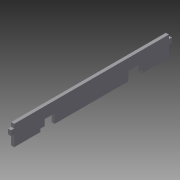
# Autodesk Inventor part: MainPanelWall3
Saved by Autodesk Inventor 2015 (Build 190159000, 159)
## iProperties
Created: 2014-08-06
Part Number: MainPanelWall3
Material: Generic
Document SubType Name: Modeling
Designer: STACKPOLE
Density: 1 g/cm^3
Appearance: Default
Author: STACKPOLE
Autodesk Inventor part; units mm, degrees
ref_plane "YZ Plane" through (0, 0, 0) normal (1, 0, 0) x (0, 1, 0)
ref_plane "XZ Plane" through (0, 0, 0) normal (0, 1, 0) x (-1, 0, 0)
ref_plane "XY Plane" through (0, 0, 0) normal (0, 0, 1) x (1, 0, 0)
sketch "Sketch1" plane through (0, 0, 0) normal (1, 0, 0) x (0, 1, 0)
  line L0 (0, 11) -> (-3, 11)
  line L1 (-3, 11) -> (-3, 16)
  line L2 (-3, 16) -> (0, 16)
  line L3 (0, 20) -> (0, 16)
  line L4 (0, 11) -> (0, 0)
  line L5 (153, 16) -> (156, 16)
  line L6 (156, 16) -> (156, 11)
  line L7 (156, 11) -> (153, 11)
  line L8 (153, 0) -> (153, 11)
  line L9 (153, 16) -> (153, 20)
  line L10 (30, 3) -> (30, 9)
  line L11 (30, 9) -> (40, 9)
  line L12 (40, 9) -> (40, 0)
  line L13 (113, 0) -> (113, 9)
  line L14 (113, 9) -> (123, 9)
  line L15 (123, 9) -> (123, 3)
  line L16 (127, 0) -> (153, 0)
  line L17 (0, 0) -> (26, 0)
  line L18 (40, 0) -> (113, 0)
  line L19 (153, 20) -> (0, 20)
  line L20 (30, 3) -> (26, 3)
  line L21 (26, 3) -> (26, 0)
  line L22 (123, 3) -> (127, 3)
  line L23 (127, 3) -> (127, 0)
  dimension "d0" = 20
  dimension "d1" = 153
  dimension "d2" = 5
  dimension "d3" = 3
  dimension "d5" = 3
  dimension "d6" = 5
  dimension "d7" = 10
  dimension "d9" = 30
  dimension "d11" = 10
  dimension "d12" = 30
  dimension "d21" = 11
  dimension "d25" = 4
  dimension "d26" = 3
  dimension "d28" = 4
  dimension "d30" = 9
  dimension "d31" = 9
  dimension "d32" = 9
  dimension "d33" = 20
  dimension "d34" = 3
  dimension "d35" = 26
  constraints: 48 end point, 25 perpendicular, 9 parallel, 4 horizontal, 2 vertical alignment, 1 horizontal alignment
  measures "d0" distance of L3.start L4.end
  measures "d1" distance of L4.end L8.start
  measures "d2" distance of L0.end L1.end
  measures "d3" distance of L0.start L0.end
  measures "d5" distance of L5.start L5.end
  measures "d6" distance of L5.end L6.end
  measures "d7" distance of L10.end L11.end
  measures "d9" distance between parallel lines of L4 L10
  measures "d11" distance of L13.end L14.end
  measures "d12" distance between parallel lines of L8 L15
  measures "d21" distance between parallel lines of L17 L0
  measures "d25" distance of L10.start L20.end
  measures "d26" distance of L17.end L20.end
  measures "d28" distance of L15.end L22.end
  measures "d30" distance between parallel lines of L17 L11
  measures "d31" distance between parallel lines of L18 L11
  measures "d32" distance between parallel lines of L14 L18
  measures "d33" distance between parallel lines of L19 L16
  measures "d34" distance of L22.end L16.start
  measures "d35" distance of L16.start L8.start
extrude "Extrusion2" add sketch "Sketch1" along normal blind 3
body "Solid2"
